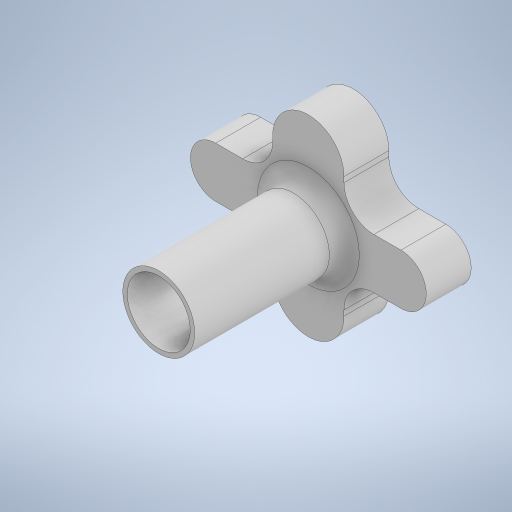
# Autodesk Inventor part: spring_extender
Saved by Autodesk Inventor 2024 (Build 280153000, 153)
## iProperties
Created: 2023-09-12
Part Number: spring_extender
Material: Generic
Document SubType Name: Modeling
Designer: Pintu
Density: 1 g/cm^3
Appearance: Default
Author: Pintu
Autodesk Inventor part; units mm, degrees
ref_plane "YZ Plane" through (0, 0, 0) normal (1, 0, 0) x (0, 1, 0)
ref_plane "XZ Plane" through (0, 0, 0) normal (0, 1, 0) x (-1, 0, 0)
ref_plane "XY Plane" through (0, 0, 0) normal (0, 0, 1) x (1, 0, 0)
sketch "Sketch1" plane through (0, 0, 0) normal (0, 0, 1) x (1, 0, 0)
  circle A0 centre (0, 0) radius 2.4
  dimension "d0" = 4.8
  constraints: 1 centre point, 1 coincident
  measures "d0" diameter of A0
extrude "Extrusion1" add sketch "Sketch1" along normal blind 10
sketch "Sketch2" plane through (0, 0, 10) normal (0, 0, 1) x (1, 0, 0)
  circle A0 centre (0, 0) radius 2.4 projected
  constraints: 1 coincident
hole "Hole1" at (0, 0, 10) direction (0, 0, -1) diameter 4.2 end through all
sketch "Sketch3" plane through (0, 0, 0) normal (0, 0, -1) x (-1, 0, 0)
  line L0 (0, 4.0429) -> (0, -4.0429) construction
  line L1 (2.3824, 4.0429) -> (2.3824, -4.0429)
  line L2 (-2.3824, -4.0429) -> (-2.3824, 4.0429)
  arc A0 (2.3824, 4.0429) -> (-2.3824, 4.0429) centre (0, 4.0429) ccw
  arc A1 (-2.3824, -4.0429) -> (2.3824, -4.0429) centre (0, -4.0429) ccw
  line L3 (6.1921, 0) -> (-6.1921, 0) construction
  line L4 (6.1921, -1.6883) -> (-6.1921, -1.6883)
  line L5 (-6.1921, 1.6883) -> (6.1921, 1.6883)
  arc A2 (6.1921, -1.6883) -> (6.1921, 1.6883) centre (6.1921, 0) ccw
  arc A3 (-6.1921, 1.6883) -> (-6.1921, -1.6883) centre (-6.1921, 0) ccw
  point P0 (0, 0)
  point P1 (2.3824, -1.6883)
  point P2 (2.3824, 1.6883)
  point P3 (-2.3824, 1.6883)
  point P4 (-2.3824, -1.6883)
  constraints: 16 end point, 8 point on circle, 8 tangent, 4 centre point, 2 midpoint, 2 parallel, 1 perpendicular, 1 vertical
extrude "Extrusion2" add sketch "Sketch3" along normal blind 3
fillet "Fillet1" radius 2 4 edges at (-2.3824, -1.6883, -1.5) (2.3824, -1.6883, -1.5) (-2.3824, 1.6883, -1.5) (2.3824, 1.6883, -1.5)
fillet "Fillet2" radius 1 1 edges at (-2.4, 0, 0)
body "Solid1"
